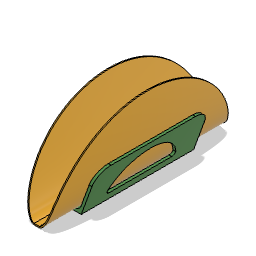
Taco Stand v11 (Autodesk Fusion 360 design; units mm, degrees)
Autodesk Fusion 360 part; units mm, degrees
note: some values were not read from the file. Set by a fixed rule: which face or edge a step refers to.
sketch "Sketch1" plane through (0, 0, 0) normal (0, 0, 1) x (1, 0, 0) in component "Taco"
sketch "Sketch2" plane through (0, 0, 0) normal (0, 0, 1) x (1, 0, 0) in component "Taco"
  line L0 (0, 0) -> (14, 0)
  line L1 (14, 0) -> (14, 58)
  line L2 (14, 58) -> (0, 58)
  line L3 (0, 58) -> (0, 0) construction
  spline S0 degree 5 poles (14, 58) (13.874869, 56.017735) (13.616265, 52.112912) (13.203338, 46.43479) (12.601895, 39.228132) (11.75815, 30.877947) (10.810105, 23.274377) (9.741015, 16.537285) (8.531582, 10.804807) (7.163405, 6.208672) (5.62372, 2.840244) (4.255736, 1.120714) (3.156063, 0.358528) (2.390725, 0.081067) (2, 0) knots 0 0 0 0 0 0 0.1 0.2 0.3 0.4 0.5 0.6 0.7 0.8 0.9 1 1 1 1 1 1
  line L4 (-14, 58) -> (0, 58)
  spline S1 degree 5 poles (-14, 58) (-13.874869, 56.017735) (-13.616265, 52.112912) (-13.203338, 46.43479) (-12.601895, 39.228132) (-11.75815, 30.877947) (-10.810105, 23.274377) (-9.741015, 16.537285) (-8.531582, 10.804807) (-7.163405, 6.208672) (-5.62372, 2.840244) (-4.255736, 1.120714) (-3.156063, 0.358528) (-2.390725, 0.081067) (-2, 0) knots 0 0 0 0 0 0 0.1 0.2 0.3 0.4 0.5 0.6 0.7 0.8 0.9 1 1 1 1 1 1
  line L5 (14.526334, 66.341717) -> (13.473666, 49.658283)
  line L6 (6.002976, 0.829684) -> (-2.002976, -0.829684)
  line L7 (-14.526334, 66.341717) -> (-13.473666, 49.658283)
  line L8 (-6.002976, 0.829684) -> (2.002976, -0.829684)
  line L9 (-14, 0) -> (-14, 58)
  line L10 (0, 0) -> (-14, 0)
  point P0 (2, 0)
  point P1 (7, 6.190427)
  point P2 (-7, 6.190427)
  dimension "d18" = 14
  dimension "d19" = 58
  dimension "d20" = 2
  constraint horizontal L0
  constraint vertical L1
  constraint horizontal L2
  constraint vertical L3
  constraint coincident L0.start L3.end
  constraint coincident L0 P0
  constraint coincident P0 S0.end
  constraint midpoint L1.end L5
  constraint midpoint P0 L6
  constraint symmetric L0.start L3 L10.start
  constraint symmetric L0.end L3 L9.start
  constraint symmetric L1.end L3 L4.start
  constraint symmetric L2.end L3 L4.end
  constraint symmetric L3 P0 S1.end
  measures "d18" distance of L0.start L0.end
  measures "d19" distance of L0.start L2.end
  measures "d20" distance of L0.start P0
extrude "Extrude1" add sketch "Sketch2" along normal mid plane 130 contours L0 L2 S0 L4 S1 L10 picked at (0, 32.93127) makes body 1 in component "Taco"
sketch "Sketch3" plane through (0, 0, 0) normal (1, 0, 0) x (0, 0, -1) in component "Taco"
  line L0 (65, 58) -> (-65, 58)
  line L1 (-65, 0) -> (-65, 58)
  line L2 (-65, 0) -> (65, 0)
  line L3 (65, 58) -> (65, 0)
  arc A0 (65, 0) -> (-65, 0) centre (0, -7.422414) ccw
  constraint tangent L0 A0
  constraint coincident L2.end L3.end
  constraint coincident L1.start L2.start
extrude "Extrude2" cut sketch "Sketch3" along normal through all and the other way through all contours L0 L3 A0 | L0 L1 A0 picked at (52.913627, 44.647437) picked at (-52.913627, 44.647437) bodies 1 in component "Taco"
shell "Shell1" thickness 0.8 removed faces 1 at (-4.656894, 57.842832, -4.532104) on bodies 1 in component "Taco"
sketch "Sketch1 (2)" plane through (0, 0, 0) normal (0, 0, 1) x (1, 0, 0) in component "Stand"
  line L0 (0, 0) -> (5.402868, 0)
  line L1 (5.402868, 0) -> (16.021942, 29.175667)
  line L2 (0, -1.875891) -> (6.7201, -1.875891)
  line L3 (6.7201, -1.875891) -> (18.021942, 29.175667)
  line L4 (16.021942, 29.175667) -> (18.021942, 29.175667)
  line L5 (0, 0) -> (0, 36.635275)
  line L6 (-5.402868, 0) -> (-16.021942, 29.175667)
  line L7 (-6.7201, -1.875891) -> (-18.021942, 29.175667)
  line L8 (-16.021942, 29.175667) -> (-18.021942, 29.175667)
  line L9 (0, 0) -> (-5.402868, 0)
  line L10 (0, -1.875891) -> (-6.7201, -1.875891)
  dimension "d27" = 70
  dimension "d29" = 2
  constraint coincident L0.start L5.start
  constraint horizontal L0
  constraint parallel L0 L2
  constraint parallel L1 L3
  constraint horizontal L4
  constraint perpendicular L0 L5
  constraint symmetric L0.start L5 L9.start
  measures "d27" angle of L0 L1
extrude "Extrude1'" add sketch "Sketch1 (2)" along normal mid plane 80 separate body contours L0 L1 L2 L3 L4 L6 L7 L8 L9 L10 picked at (-10.048303, 9.099925) makes body 2 in component "Stand"
sketch "Sketch2 (2)" plane through (0, 0, 0) normal (1, 0, 0) x (0, 0, -1) in component "Stand"
  line L0 (40, 29.175667) -> (-40, 29.175667)
  line L1 (-40, 29.175667) -> (-40, -1.875891)
  line L2 (-40, -1.875891) -> (40, -1.875891)
  line L3 (40, -1.875891) -> (40, 29.175667)
  line L4 (0, 29.175667) -> (0, -1.875891) construction
  line L5 (25, 23.649888) -> (-25, 23.649888)
  line L6 (-25, 23.649888) -> (-25, 3.649888)
  line L7 (-25, 3.649888) -> (25, 3.649888)
  line L8 (25, 3.649888) -> (25, 23.649888)
  line L9 (25, 23.649888) -> (-25, 3.649888) construction
  line L10 (-25, 23.649888) -> (25, 3.649888) construction
  arc A0 (25, 3.649888) -> (-25, 3.649888) centre (0, -1.975112) ccw
  point P0 (0, 13.649888)
  dimension "d32" = 50
  dimension "d33" = 20
  constraint horizontal L5
  constraint perpendicular L5 L6
  constraint parallel L5 L7
  constraint parallel L6 L8
extrude "Extrude2'" cut sketch "Sketch2 (2)" along normal through all and the other way through all contours L7 A0 picked at (5.820532, 8.026406) bodies 2 in component "Stand"
fillet "Fillet1" radius 10 4 edges at (-17.021942, 29.175667, -40) (17.021942, 29.175667, -40) (17.021942, 29.175667, 40) (-17.021942, 29.175667, 40) on bodies 2 in component "Stand"
fillet "Fillet2" radius 2 4 edges at (-7.731319, 3.649888, 25) (-7.731319, 3.649888, -25) (7.731319, 3.649888, 25) (7.731319, 3.649888, -25) on bodies 2 in component "Stand"
fillet "Fillet3" radius 5 2 edges at (5.402868, 0, 0) (-5.402868, 0, 0) on bodies 2 in component "Stand"
component "Taco" placed x (1, 0, 0) y (0, 1, 0) z (0, 0, 1) at (0, 0, 0)
component "Stand" placed x (1, 0, 0) y (0, 1, 0) z (0, 0, 1) at (0, 0, 0)
equation "d21 = ( 130 / 2 ) * 1 mm"
